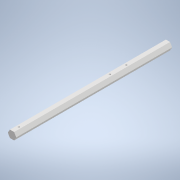
# Autodesk Inventor part: Eje_Salida
Saved by Autodesk Inventor 2022 (Build 260153000, 153)
## iProperties
Created: 2022-02-21
Part Number: Eje_Salida
Material: Generic
Document SubType Name: Modeling
Designer: katha
Density: 1 g/cm^3
Appearance: Default
Author: katha
Autodesk Inventor part; units mm, degrees
ref_plane "YZ Plane" through (0, 0, 0) normal (1, 0, 0) x (0, 1, 0)
ref_plane "XZ Plane" through (0, 0, 0) normal (0, 1, 0) x (-1, 0, 0)
ref_plane "XY Plane" through (0, 0, 0) normal (0, 0, 1) x (1, 0, 0)
sketch "Sketch4" plane through (0, 0, 0) normal (0, 0, 1) x (1, 0, 0)
  line L0 (0, 0) -> (3.1, 0) construction
  circle A0 centre (0, 0) radius 3.1 construction
  line L1 (0, 0) -> (1.55, 2.6847) construction
  line L2 (0, 0) -> (-1.55, 2.6847) construction
  line L3 (0, 0) -> (-3.1, 0) construction
  line L4 (0, 0) -> (-1.55, -2.6847) construction
  line L5 (0, 0) -> (1.55, -2.6847) construction
  line L6 (-1.55, 2.6847) -> (1.55, 2.6847)
  line L7 (1.55, 2.6847) -> (3.1, 0)
  line L8 (3.1, 0) -> (1.55, -2.6847)
  line L9 (1.55, -2.6847) -> (-1.55, -2.6847)
  line L10 (-1.55, -2.6847) -> (-3.1, 0)
  line L11 (-3.1, 0) -> (-1.55, 2.6847)
  dimension "d21" = 3.1
  dimension "d24" = 360
  constraints: 24 end point, 3 parallel, 2 horizontal, 1 coincident, 1 horizontal alignment, 21 other
  measures "d21" distance of L0.start L0.end
extrude "Extrusion6" add sketch "Sketch4" along normal blind 115
sketch "Sketch5" plane through (-1.55, 2.6847, 0) normal (0, 1, 0) x (1, 0, 0)
  line L0 (3.1, -115) -> (0, -115) projected
  line L1 (3.1, 0) -> (0, 0) construction
  line L2 (0, -115) -> (3.1, -115) projected
  line L3 (1.55, -115) -> (1.55, 0) construction
  circle A0 centre (1.55, -30.9) radius 0.65
  circle A1 centre (1.55, -42.9) radius 0.65
  circle A2 centre (1.55, -110) radius 0.65
  line L4 (9.05, -74) -> (-5.95, -74)
  line L5 (-5.95, -80) -> (9.05, -80)
  line L6 (9.05, 0) -> (-5.95, 0)
  dimension "d28" = 1.3
  dimension "d29" = 84.1
  dimension "d30" = 72.1
  dimension "d31" = 5
  constraints: 8 end point, 3 centre point, 3 horizontal, 3 point on line, 2 equal radius, 1 midpoint, 1 perpendicular, 6 other
  measures "d28" diameter of A0
  measures "d29" distance from line of A0.centre L0
  measures "d30" distance from line of A1.centre L0
  measures "d31" distance from line of A2.centre L0
extrude "Extrusion7" cut sketch "Sketch5" against normal blind 6
body "Solid2"
